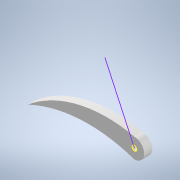
# Autodesk Inventor part: бровь
Saved by Autodesk Inventor 2020 (Build 240168000, 168)
## iProperties
Created: 2022-02-27
Part Number: бровь
Material: Типовые
Document SubType Name: Modeling
Designer: Администратор
Density: 1 g/cm^3
Appearance: По умолчанию
Author: Администратор
Autodesk Inventor part; units mm, degrees
ref_plane "YZ Plane" through (0, 0, 0) normal (1, 0, 0) x (0, 1, 0)
ref_plane "XZ Plane" through (0, 0, 0) normal (0, 1, 0) x (-1, 0, 0)
ref_plane "XY Plane" through (0, 0, 0) normal (0, 0, 1) x (1, 0, 0)
sketch "Эскиз1" plane through (0, 0, 0) normal (0, 0, 1) x (1, 0, 0)
  circle A0 centre (0, 0) radius 1.5
  circle A1 centre (0, 0) radius 6.013
  arc A2 (0, 6.013) -> (-65.094, -9.612) centre (-16.742, -67.6435) ccw
  arc A3 (0, -6.013) -> (-65.094, -9.612) centre (-28.1526, -87.2929) ccw
  dimension "d0" = 3
  constraints: 6 point on circle, 4 centre point, 2 coincident
  measures "d0" diameter of A0
extrude "Выдавливание1" add sketch "Эскиз1" along normal blind 5 contours A1 A3 | A1 A3 A2 picked at (-3.7216, -2.4926)
sketch "Эскиз2" plane through (0, 0, 5) normal (0, 0, 1) x (1, 0, 0)
  circle A0 centre (0, 0) radius 1.5 projected
  circle A1 centre (0, 0) radius 1.5 projected
  line L0 (0, 0) -> (-18.0245, 38.8961)
  constraints: 2 end point
